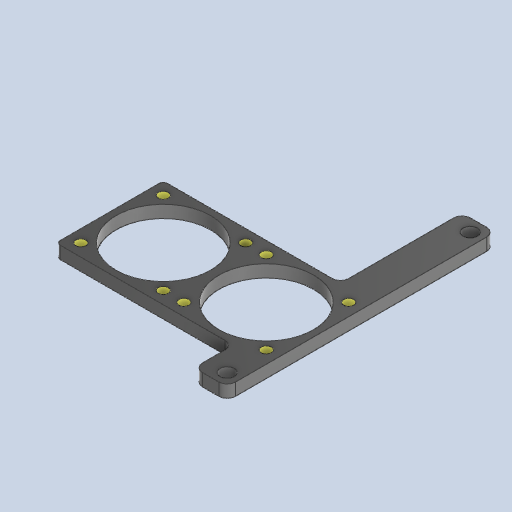
# Autodesk Inventor part: MainBoard_fan_plate
Saved by Autodesk Inventor 2022 (Build 260153000, 153)
## iProperties
Created: 2022-07-04
Part Number: MainBoard_fan_plate
Material: 一般
Document SubType Name: Modeling
Designer: Masato Kubotera
Density: 1 g/cm^3
Appearance: 滑らか - 黒
Description: PLA
Mass: 2.23917 g
Surface Area: 28.5876 cm^2
Volume: 2.23917 cm^3
Author: Masato Kubotera
Autodesk Inventor part; units mm, degrees
ref_plane "YZ Plane" through (0, 0, 0) normal (1, 0, 0) x (0, 1, 0)
ref_plane "XZ Plane" through (0, 0, 0) normal (0, 1, 0) x (-1, 0, 0)
derived "MainBoard.ipt"
sketch "スケッチ3" plane through (0, 0, -88.5) normal (0, 0, 1) x (1, 0, 0)
  line L0 (20.25, -135) -> (20.25, 0)
  line L1 (-83.25, 0) -> (-83.25, -135)
  line L2 (-31.5, -135) -> (-31.5, 0) construction
  line L3 (-83.25, -67.5) -> (20.25, -67.5) construction
  line L4 (-56.5, 1.4849) -> (-56.5, 5)
  line L5 (-56.5, 5) -> (-6.5, 5)
  line L6 (-6.5, 5) -> (-6.5, 1.4849)
  arc A0 (-57.9849, 0) -> (-56.5, 1.4849) centre (-57.2425, 0.7425) ccw
  arc A1 (-6.5, 1.4849) -> (-5.0151, 0) centre (-5.7575, 0.7425) ccw
  line L7 (-57.9849, 0) -> (-83.25, 0)
  line L8 (20.25, 0) -> (-5.0151, 0)
  line L9 (-6.5, 0) -> (-56.5, 0)
  line L10 (-56.5, -136.4849) -> (-56.5, -140)
  line L11 (-56.5, -140) -> (-6.5, -140)
  line L12 (-6.5, -140) -> (-6.5, -136.4849)
  arc A2 (-56.5, -136.4849) -> (-57.9849, -135) centre (-57.2425, -135.7425) ccw
  arc A3 (-5.0151, -135) -> (-6.5, -136.4849) centre (-5.7575, -135.7425) ccw
  line L13 (-57.9849, -135) -> (-83.25, -135)
  line L14 (20.25, -135) -> (-5.0151, -135)
  line L15 (-6.5, -135) -> (-56.5, -135)
  line L16 (18, -127.5) -> (-47, -127.5) construction
  line L17 (-47, -127.5) -> (-47, -7.5) construction
  line L18 (-47, -7.5) -> (18, -7.5) construction
  line L19 (18, -7.5) -> (18, -127.5) construction
  line L20 (18, -127.5) -> (-47, -7.5) construction
  line L21 (-47, -127.5) -> (18, -7.5) construction
  line L22 (-46, -116.5) -> (-46, -18.5)
  line L23 (-36.0627, -9.5) -> (7.0627, -9.5)
  line L24 (15, -10.5) -> (-44, -10.5) construction
  line L25 (-44, -10.5) -> (-44, -124.5) construction
  line L26 (-44, -124.5) -> (15, -124.5) construction
  line L27 (15, -124.5) -> (15, -10.5) construction
  line L28 (15, -10.5) -> (-44, -124.5) construction
  line L29 (-44, -10.5) -> (15, -124.5) construction
  circle A4 centre (15, -10.5) radius 2
  circle A5 centre (-44, -10.5) radius 2
  arc A6 (-44, -16.5) -> (-38.0471, -11.25) centre (-44, -10.5) ccw
  arc A7 (9.0471, -11.25) -> (15, -16.5) centre (15, -10.5) ccw
  line L30 (17, -18.5) -> (17, -116.5)
  line L31 (-14.5, -7.5) -> (-14.5, -127.5) construction
  line L32 (-76.25, -65) -> (-54, -65)
  line L33 (-52, -63) -> (-52, -7)
  line L34 (-54, -5) -> (-76.25, -5)
  line L35 (-78.25, -7) -> (-78.25, -63)
  arc A8 (-78.25, -63) -> (-76.25, -65) centre (-76.25, -63) ccw
  arc A9 (-54, -65) -> (-52, -63) centre (-54, -63) ccw
  arc A10 (-52, -7) -> (-54, -5) centre (-54, -7) ccw
  arc A11 (-76.25, -5) -> (-78.25, -7) centre (-76.25, -7) ccw
  arc A12 (-44, -16.5) -> (-46, -18.5) centre (-44, -18.5) ccw
  arc A13 (-36.0627, -9.5) -> (-38.0471, -11.25) centre (-36.0627, -11.5) ccw
  arc A14 (9.0471, -11.25) -> (7.0627, -9.5) centre (7.0627, -11.5) ccw
  arc A15 (17, -18.5) -> (15, -16.5) centre (15, -18.5) ccw
  line L36 (-36.0627, -125.5) -> (7.0627, -125.5)
  circle A16 centre (15, -124.5) radius 2
  circle A17 centre (-44, -124.5) radius 2
  arc A18 (-38.0471, -123.75) -> (-44, -118.5) centre (-44, -124.5) ccw
  arc A19 (15, -118.5) -> (9.0471, -123.75) centre (15, -124.5) ccw
  line L37 (-76.25, -70) -> (-54, -70)
  line L38 (-52, -72) -> (-52, -128)
  line L39 (-54, -130) -> (-76.25, -130)
  line L40 (-78.25, -128) -> (-78.25, -72)
  arc A20 (-76.25, -70) -> (-78.25, -72) centre (-76.25, -72) ccw
  arc A21 (-52, -72) -> (-54, -70) centre (-54, -72) ccw
  arc A22 (-54, -130) -> (-52, -128) centre (-54, -128) ccw
  arc A23 (-78.25, -128) -> (-76.25, -130) centre (-76.25, -128) ccw
  arc A24 (-46, -116.5) -> (-44, -118.5) centre (-44, -116.5) ccw
  arc A25 (-38.0471, -123.75) -> (-36.0627, -125.5) centre (-36.0627, -123.5) ccw
  arc A26 (7.0627, -125.5) -> (9.0471, -123.75) centre (7.0627, -123.5) ccw
  arc A27 (15, -118.5) -> (17, -116.5) centre (15, -116.5) ccw
  point P0 (0, 0)
  point P1 (-31.5, -67.5)
  point P2 (-56.5, 0)
  point P3 (-14.5, -67.5)
  point P4 (-46, -16.1569)
  point P5 (-38.0839, -9.5)
  point P6 (9.0839, -9.5)
  point P7 (17, -16.1569)
ref_plane "作業平面1" through (20.25, 0, -88.5) normal (0, 0, 1) x (-1, 0, 0)
sketch "スケッチ2" plane through (20.25, 0, -88.5) normal (0, 0, 1) x (-1, 0, 0)
  line L0 (4.25, 7.5) -> (65.25, 7.5)
  line L1 (67.25, 9.5) -> (67.25, 13.5)
  line L2 (65.25, 15.5) -> (39.75, 15.5)
  line L3 (37.75, 17.5) -> (37.75, 57.5)
  line L4 (36.75, 58.5) -> (12.75, 58.5)
  line L5 (2.25, 13.5) -> (2.25, 9.5)
  line L6 (37.25, 8) -> (12.25, 8) construction
  line L7 (12.25, 8) -> (12.25, 33) construction
  line L8 (12.25, 33) -> (37.25, 33) construction
  line L9 (37.25, 33) -> (37.25, 8) construction
  line L10 (37.25, 8) -> (12.25, 33) construction
  line L11 (12.25, 8) -> (37.25, 33) construction
  line L12 (14.75, 10.5) -> (34.75, 10.5) construction
  line L13 (34.75, 10.5) -> (34.75, 30.5) construction
  line L14 (34.75, 30.5) -> (14.75, 30.5) construction
  line L15 (14.75, 30.5) -> (14.75, 10.5) construction
  line L16 (14.75, 10.5) -> (34.75, 30.5) construction
  line L17 (34.75, 10.5) -> (14.75, 30.5) construction
  circle A0 centre (14.75, 10.5) radius 1.25
  circle A1 centre (34.75, 10.5) radius 1.25
  circle A2 centre (14.75, 30.5) radius 1.25
  circle A3 centre (34.75, 30.5) radius 1.25
  circle A4 centre (5.25, 10.5) radius 3
  circle A5 centre (64.25, 10.5) radius 3
  circle A6 centre (64.25, 10.5) radius 1.75
  circle A7 centre (5.25, 10.5) radius 1.75
  line L18 (2.25, 7.5) -> (2.25, 127.5) construction
  line L19 (67.25, 7.5) -> (2.25, 7.5) construction
  line L20 (67.25, 127.5) -> (67.25, 7.5) construction
  line L21 (4.25, 15.5) -> (9.75, 15.5)
  line L22 (11.75, 17.5) -> (11.75, 57.5)
  circle A8 centre (14.75, 35.5) radius 1.25
  line L23 (37.25, 33) -> (12.25, 33) construction
  line L24 (12.25, 33) -> (12.25, 58) construction
  line L25 (12.25, 58) -> (37.25, 58) construction
  circle A9 centre (14.75, 55.5) radius 1.25
  circle A10 centre (34.75, 55.5) radius 1.25
  line L26 (37.25, 58) -> (37.25, 33) construction
  circle A11 centre (34.75, 35.5) radius 1.25
  circle A12 centre (24.75, 20.5) radius 11.5
  circle A13 centre (24.75, 45.5) radius 11.5
  arc A14 (9.75, 15.5) -> (11.75, 17.5) centre (9.75, 17.5) ccw
  arc A15 (37.75, 17.5) -> (39.75, 15.5) centre (39.75, 17.5) ccw
  arc A16 (4.25, 15.5) -> (2.25, 13.5) centre (4.25, 13.5) ccw
  arc A17 (67.25, 13.5) -> (65.25, 15.5) centre (65.25, 13.5) ccw
  arc A18 (12.75, 58.5) -> (11.75, 57.5) centre (12.75, 57.5) ccw
  arc A19 (37.75, 57.5) -> (36.75, 58.5) centre (36.75, 57.5) ccw
  arc A20 (2.25, 9.5) -> (4.25, 7.5) centre (4.25, 9.5) ccw
  arc A21 (65.25, 7.5) -> (67.25, 9.5) centre (65.25, 9.5) ccw
  point P0 (20.25, 0)
  point P1 (67.25, 7.5)
  point P2 (2.25, 7.5)
  point P3 (2.25, 15.5)
  point P4 (64.25, 7.5)
  point P5 (67.25, 10.5)
  dimension "d1" = 25
  dimension "d2" = 20
  dimension "d3" = 20
  dimension "d4" = 2.5
  dimension "d7" = 20
  dimension "d10" = 20
  dimension "d13" = 0.5
  dimension "d14" = 6
  dimension "d15" = 6
  dimension "d16" = 3.5
  dimension "d17" = 3.5
  dimension "d18" = 10
  dimension "d19" = 25
  dimension "d20" = 8
  dimension "d23" = 25
  dimension "d28" = 23
  dimension "d29" = 0.5
  dimension "d30" = 0.5
  dimension "d31" = 0.5
  dimension "d34" = 25
  dimension "d39" = 2
  dimension "d40" = 2
  dimension "d41" = 1
  dimension "d44" = 2
  constraints: 48 end point, 22 centre point, 16 point on circle, 16 tangent, 9 perpendicular, 8 point on line, 6 coincident, 5 collinear, 4 equal radius, 4 horizontal, 4 midpoint, 4 parallel, 3 vertical, 23 other
  measures "d1" distance of L7.end L8.end
  measures "d2" distance of L14.end L13.end
  measures "d3" distance of L13.end L12.end
  measures "d4" diameter of A0
  measures "d7" distance of A0.centre A1.centre
  measures "d10" distance of A0.centre A2.centre
  measures "d13" vertical distance of point (2.25, 7.5) L6.end
  measures "d14" diameter of A4
  measures "d15" diameter of A5
  measures "d16" diameter of A6
  measures "d17" diameter of A7
  measures "d18" distance between parallel lines of L7 L5
  measures "d19" distance of L8.end L6.start
  measures "d20" distance between parallel lines of L0 L21
  measures "d23" distance of A0.centre A8.centre
  measures "d28" diameter of A12
  measures "d29" distance between parallel lines of L22 L7
  measures "d30" distance between parallel lines of L3 L9
  measures "d31" distance between parallel lines of L4 L25
  measures "d34" distance of A12.centre A13.centre
  measures "d39" radius of A14
  measures "d40" radius of A16
  measures "d41" radius of A18
  measures "d44" radius of A20
extrude "押し出し1" add sketch "スケッチ2" along normal blind 3
equation "\"d7\" = d2"
equation "\"d10\" = d3"
equation "\"d23\" = d19"
equation "\"d30\" = d29"
equation "\"d31\" = d29"
equation "\"d34\" = d23"
